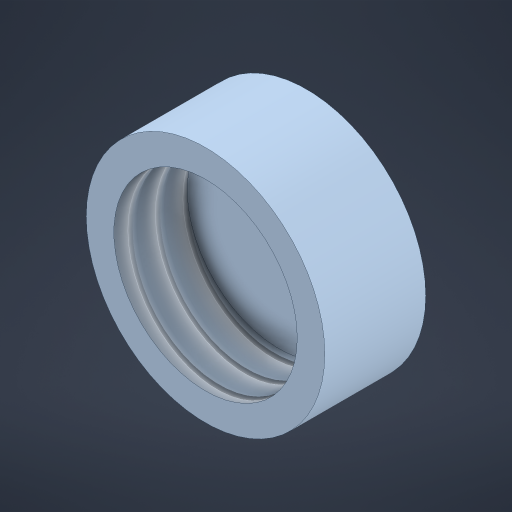
# Autodesk Inventor part: TOP STOPPER
Saved by Autodesk Inventor 2023 (Build 270158000, 158)
## iProperties
Created: 2023-12-28
Part Number: TOP STOPPER
Material: Steel, Alloy
Document SubType Name: Modeling
Designer: User
Density: 7.73 g/cm^3
Appearance: Light Steel Blue
Author: User
Autodesk Inventor part; units mm, degrees
ref_plane "YZ Plane" through (0, 0, 0) normal (1, 0, 0) x (0, 1, 0)
ref_plane "XZ Plane" through (0, 0, 0) normal (0, 1, 0) x (-1, 0, 0)
ref_plane "XY Plane" through (0, 0, 0) normal (0, 0, 1) x (1, 0, 0)
sketch "Sketch1" plane through (0, 0, 0) normal (0, 0, 1) x (1, 0, 0)
  circle A0 centre (0, 0) radius 6.5
  dimension "d0" = 13
  constraints: 1 centre point, 1 coincident
  measures "d0" diameter of A0
extrude "Extrusion1" add sketch "Sketch1" along normal blind 5.5
sketch "Sketch2" plane through (0, 0, 5.5) normal (0, 0, 1) x (1, 0, 0)
  circle A0 centre (0, 0) radius 6.5 projected
  constraints: 1 coincident
hole "Hole1" at (0, 0, 5.5) direction (0, 0, -1) diameter 10 depth 4
thread "Thread1" size "M10x1.5" class "6H" standard "ANSI Metric M Profile" length 4
body "Solid1"
